Autodesk Inventor part; units mm, degrees
(part 2 of 2)
sketch "Эскиз17" plane through (97.4, -95.275, 2.1) normal (1, 0, 0) x (0, 0, -1)
  line L0 (-33.4467, 33.4271) -> (-33.4467, 22.4297) construction
  line L1 (-33.4467, 22.4297) -> (-36.1893, 22.4297) construction
  line L2 (-36.1893, 22.4297) -> (-36.1893, 33.4271) construction
  line L3 (-36.1893, 33.4271) -> (-33.4467, 33.4271) construction
  line L4 (-30.2454, 64.7817) -> (-30.2454, 44.3238) construction
  line L5 (-30.2454, 44.3238) -> (-33.7846, 44.3238) construction
  line L6 (-33.7846, 44.3238) -> (-33.7846, 64.7817) construction
  line L7 (-33.7846, 64.7817) -> (-30.2454, 64.7817) construction
  spline S0 degree 2 poles (-31.5525, 64.6293) (-31.1714, 64.6293) (-30.9123, 64.515) knots 0 0 0 1 1 1
  spline S1 degree 2 poles (-30.9123, 64.515) (-30.7218, 64.4292) (-30.4169, 64.1339) (-30.3445, 63.9586) knots 0 0 0 1 2 2 2
  spline S2 degree 2 poles (-30.3445, 63.9586) (-30.2454, 63.7261) (-30.2454, 63.4193) knots 0 0 0 1 1 1
  spline S3 degree 2 poles (-30.2454, 63.4193) (-30.2454, 62.8667) (-30.9314, 62.2036) (-31.5411, 62.2036) knots 0 0 0 1 2 2 2
  spline S4 degree 2 poles (-31.5411, 62.2036) (-32.1452, 62.2036) (-32.8292, 62.8629) (-32.8292, 63.4136) knots 0 0 0 1 2 2 2
  spline S5 degree 2 poles (-32.8292, 63.4136) (-32.8292, 63.97) (-32.149, 64.6293) (-31.5525, 64.6293) knots 0 0 0 1 2 2 2
  spline S6 degree 2 poles (-31.5354, 64.1091) (-31.9603, 64.1091) (-32.3986, 63.7166) (-32.3986, 63.4136) knots 0 0 0 1 2 2 2
  spline S7 degree 2 poles (-32.3986, 63.4136) (-32.3986, 63.1106) (-31.9641, 62.7238) (-31.5297, 62.7238) knots 0 0 0 1 2 2 2
  spline S8 degree 2 poles (-31.5297, 62.7238) (-31.099, 62.7238) (-30.676, 63.1011) (-30.676, 63.4136) knots 0 0 0 1 2 2 2
  spline S9 degree 2 poles (-30.676, 63.4136) (-30.676, 63.7261) (-31.1048, 64.1091) (-31.5354, 64.1091) knots 0 0 0 1 2 2 2
  line L8 (-30.9752, 61.8282) -> (-30.9752, 61.3804)
  line L9 (-30.9752, 61.3804) -> (-31.242, 61.3804)
  spline S10 degree 2 poles (-31.242, 61.3804) (-31.1048, 61.2928) (-30.9352, 60.9974) (-30.9352, 60.8164) knots 0 0 0 1 2 2 2
  spline S11 degree 2 poles (-30.9352, 60.8164) (-30.9352, 60.5001) (-31.4287, 60.0599) (-31.8708, 60.0599) knots 0 0 0 1 2 2 2
  spline S12 degree 2 poles (-31.8708, 60.0599) (-32.3243, 60.0599) (-32.8273, 60.5039) (-32.8273, 60.8183) knots 0 0 0 1 2 2 2
  spline S13 degree 2 poles (-32.8273, 60.8183) (-32.8273, 60.9688) (-32.7073, 61.2127) (-32.5625, 61.348) knots 0 0 0 1 2 2 2
  line L10 (-32.5625, 61.348) -> (-33.4771, 61.348)
  line L11 (-33.4771, 61.348) -> (-33.4771, 61.8282)
  line L12 (-33.4771, 61.8282) -> (-30.9752, 61.8282)
  spline S14 degree 2 poles (-31.8498, 61.3557) (-32.1547, 61.3557) (-32.4462, 61.1118) (-32.4462, 60.9384) knots 0 0 0 1 2 2 2
  spline S15 degree 2 poles (-32.4462, 60.9384) (-32.4462, 60.7707) (-32.1795, 60.5477) (-31.8746, 60.5477) knots 0 0 0 1 2 2 2
  spline S16 degree 2 poles (-31.8746, 60.5477) (-31.5907, 60.5477) (-31.3144, 60.7764) (-31.3144, 60.946) knots 0 0 0 1 2 2 2
  spline S17 degree 2 poles (-31.3144, 60.946) (-31.3144, 61.1232) (-31.5849, 61.3557) (-31.8498, 61.3557) knots 0 0 0 1 2 2 2
  line L13 (-32.7873, 59.6788) -> (-30.9752, 59.6788)
  line L14 (-30.9752, 59.6788) -> (-30.9752, 59.1986)
  line L15 (-30.9752, 59.1986) -> (-32.7873, 59.1986)
  line L16 (-32.7873, 59.1986) -> (-32.7873, 59.6788)
  line L17 (-30.7313, 59.6788) -> (-30.2873, 59.6788)
  line L18 (-30.2873, 59.6788) -> (-30.2873, 59.1986)
  line L19 (-30.2873, 59.1986) -> (-30.7313, 59.1986)
  line L20 (-30.7313, 59.1986) -> (-30.7313, 59.6788)
  line L21 (-31.5106, 57.1331) -> (-31.5964, 57.6057)
  spline S18 degree 2 poles (-31.5964, 57.6057) (-31.4554, 57.6285) (-31.3125, 57.7981) (-31.3125, 57.9334) knots 0 0 0 1 2 2 2
  spline S19 degree 2 poles (-31.3125, 57.9334) (-31.3125, 58.1106) (-31.5602, 58.324) (-31.8498, 58.324) knots 0 0 0 1 2 2 2
  spline S20 degree 2 poles (-31.8498, 58.324) (-32.1718, 58.324) (-32.4367, 58.1068) (-32.4367, 57.9258) knots 0 0 0 1 2 2 2
  spline S21 degree 2 poles (-32.4367, 57.9258) (-32.4367, 57.7886) (-32.2804, 57.6152) (-32.0918, 57.579) knots 0 0 0 1 2 2 2
  line L22 (-32.0918, 57.579) -> (-32.1718, 57.1083)
  spline S22 degree 2 poles (-32.1718, 57.1083) (-32.4958, 57.1807) (-32.8273, 57.598) (-32.8273, 57.9467) knots 0 0 0 1 2 2 2
  spline S23 degree 2 poles (-32.8273, 57.9467) (-32.8273, 58.3431) (-32.3262, 58.8156) (-31.8822, 58.8156) knots 0 0 0 1 2 2 2
  spline S24 degree 2 poles (-31.8822, 58.8156) (-31.4344, 58.8156) (-30.9352, 58.3431) (-30.9352, 57.9391) knots 0 0 0 1 2 2 2
  spline S25 degree 2 poles (-30.9352, 57.9391) (-30.9352, 57.6076) (-31.2191, 57.2188) (-31.5106, 57.1331) knots 0 0 0 1 2 2 2
  line L23 (-31.5278, 56.4109) -> (-31.4496, 56.8454)
  spline S26 degree 2 poles (-31.4496, 56.8454) (-31.1867, 56.7711) (-30.9352, 56.4128) (-30.9352, 56.0603) knots 0 0 0 1 2 2 2
  spline S27 degree 2 poles (-30.9352, 56.0603) (-30.9352, 55.7383) (-31.0876, 55.4239) (-31.3201, 55.2962) (-31.6326, 55.2962) knots 0 0 0 1 2 3 3 3
  line L24 (-31.6326, 55.2962) -> (-32.1928, 55.3038)
  spline S28 degree 2 poles (-32.1928, 55.3038) (-32.431, 55.3038) (-32.6577, 55.2581) (-32.7873, 55.1952) knots 0 0 0 1 2 2 2
  line L25 (-32.7873, 55.1952) -> (-32.7873, 55.6697)
  spline S29 degree 2 poles (-32.7873, 55.6697) (-32.7397, 55.6887) (-32.6463, 55.7154) knots 0 0 0 1 1 1
  spline S30 degree 2 poles (-32.6463, 55.7154) (-32.6025, 55.7268) (-32.5891, 55.7326) knots 0 0 0 1 1 1
  spline S31 degree 2 poles (-32.5891, 55.7326) (-32.7073, 55.8545) (-32.8273, 56.1346) (-32.8273, 56.2928) knots 0 0 0 1 2 2 2
  spline S32 degree 2 poles (-32.8273, 56.2928) (-32.8273, 56.5729) (-32.5243, 56.8949) (-32.2919, 56.8949) knots 0 0 0 1 2 2 2
  spline S33 degree 2 poles (-32.2919, 56.8949) (-32.1375, 56.8949) (-31.8974, 56.7482) (-31.7698, 56.4833) (-31.7221, 56.2337) knots 0 0 0 1 2 3 3 3
  spline S34 degree 2 poles (-31.7221, 56.2337) (-31.6593, 55.8983) (-31.604, 55.7688) knots 0 0 0 1 1 1
  line L26 (-31.604, 55.7688) -> (-31.5564, 55.7688)
  spline S35 degree 2 poles (-31.5564, 55.7688) (-31.4192, 55.7688) (-31.301, 55.906) (-31.301, 56.0946) knots 0 0 0 1 2 2 2
  spline S36 degree 2 poles (-31.301, 56.0946) (-31.301, 56.2223) (-31.402, 56.3671) (-31.5278, 56.4109) knots 0 0 0 1 2 2 2
  spline S37 degree 2 poles (-31.9165, 55.7688) (-31.947, 55.8602) (-32.0327, 56.2604) (-32.0727, 56.3214) knots 0 0 0 1 2 2 2
  spline S38 degree 2 poles (-32.0727, 56.3214) (-32.1394, 56.4147) (-32.2423, 56.4147) knots 0 0 0 1 1 1
  spline S39 degree 2 poles (-32.2423, 56.4147) (-32.3433, 56.4147) (-32.49, 56.2642) (-32.49, 56.148) knots 0 0 0 1 2 2 2
  spline S40 degree 2 poles (-32.49, 56.148) (-32.49, 56.0184) (-32.4043, 55.9022) knots 0 0 0 1 1 1
  spline S41 degree 2 poles (-32.4043, 55.9022) (-32.3395, 55.8145) (-32.2461, 55.7878) knots 0 0 0 1 1 1
  spline S42 degree 2 poles (-32.2461, 55.7878) (-32.1852, 55.7688) (-32.0118, 55.7688) knots 0 0 0 1 1 1
  line L27 (-32.0118, 55.7688) -> (-31.9165, 55.7688)
  line L28 (-32.7873, 54.8256) -> (-30.2873, 54.8256)
  line L29 (-30.2873, 54.8256) -> (-30.2873, 54.3454)
  line L30 (-30.2873, 54.3454) -> (-32.7873, 54.3454)
  line L31 (-32.7873, 54.3454) -> (-32.7873, 54.8256)
  line L32 (-32.7873, 52.8858) -> (-30.9752, 52.8858)
  line L33 (-30.9752, 52.8858) -> (-30.9752, 52.4056)
  line L34 (-30.9752, 52.4056) -> (-32.7873, 52.4056)
  line L35 (-32.7873, 52.4056) -> (-32.7873, 52.8858)
  line L36 (-30.7313, 52.8858) -> (-30.2873, 52.8858)
  line L37 (-30.2873, 52.8858) -> (-30.2873, 52.4056)
  line L38 (-30.2873, 52.4056) -> (-30.7313, 52.4056)
  line L39 (-30.7313, 52.4056) -> (-30.7313, 52.8858)
  line L40 (-32.7873, 50.2695) -> (-32.7873, 50.7497)
  line L41 (-32.7873, 50.7497) -> (-31.8631, 50.7497)
  spline S43 degree 2 poles (-31.8631, 50.7497) (-31.5697, 50.7497) (-31.3963, 50.8107) (-31.301, 50.9498) (-31.301, 51.047) knots 0 0 0 1 2 3 3 3
  spline S44 degree 2 poles (-31.301, 51.047) (-31.301, 51.1708) (-31.4382, 51.369) (-31.6631, 51.4414) (-31.966, 51.4414) knots 0 0 0 1 2 3 3 3
  line L42 (-31.966, 51.4414) -> (-32.7873, 51.4414)
  line L43 (-32.7873, 51.4414) -> (-32.7873, 51.9216)
  line L44 (-32.7873, 51.9216) -> (-30.9752, 51.9216)
  line L45 (-30.9752, 51.9216) -> (-30.9752, 51.4757)
  line L46 (-30.9752, 51.4757) -> (-31.242, 51.4757)
  spline S45 degree 2 poles (-31.242, 51.4757) (-30.9352, 51.2394) (-30.9352, 50.8793) knots 0 0 0 1 1 1
  spline S46 degree 2 poles (-30.9352, 50.8793) (-30.9352, 50.7192) (-31.0495, 50.4563) (-31.2267, 50.3229) (-31.4516, 50.2695) (-31.6612, 50.2695) knots 0 0 0 1 2 3 4 4 4
  line L47 (-31.6612, 50.2695) -> (-32.7873, 50.2695)
  line L48 (-30.9752, 49.797) -> (-30.9752, 49.3492)
  line L49 (-30.9752, 49.3492) -> (-31.242, 49.3492)
  spline S47 degree 2 poles (-31.242, 49.3492) (-31.1048, 49.2615) (-30.9352, 48.9662) (-30.9352, 48.7852) knots 0 0 0 1 2 2 2
  spline S48 degree 2 poles (-30.9352, 48.7852) (-30.9352, 48.4688) (-31.4287, 48.0287) (-31.8708, 48.0287) knots 0 0 0 1 2 2 2
  spline S49 degree 2 poles (-31.8708, 48.0287) (-32.3243, 48.0287) (-32.8273, 48.4727) (-32.8273, 48.7871) knots 0 0 0 1 2 2 2
  spline S50 degree 2 poles (-32.8273, 48.7871) (-32.8273, 48.9376) (-32.7073, 49.1815) (-32.5625, 49.3168) knots 0 0 0 1 2 2 2
  line L50 (-32.5625, 49.3168) -> (-33.4771, 49.3168)
  line L51 (-33.4771, 49.3168) -> (-33.4771, 49.797)
  line L52 (-33.4771, 49.797) -> (-30.9752, 49.797)
  spline S51 degree 2 poles (-31.8498, 49.3244) (-32.1547, 49.3244) (-32.4462, 49.0805) (-32.4462, 48.9071) knots 0 0 0 1 2 2 2
  spline S52 degree 2 poles (-32.4462, 48.9071) (-32.4462, 48.7394) (-32.1795, 48.5165) (-31.8746, 48.5165) knots 0 0 0 1 2 2 2
  spline S53 degree 2 poles (-31.8746, 48.5165) (-31.5907, 48.5165) (-31.3144, 48.7451) (-31.3144, 48.9147) knots 0 0 0 1 2 2 2
  spline S54 degree 2 poles (-31.3144, 48.9147) (-31.3144, 49.0919) (-31.5849, 49.3244) (-31.8498, 49.3244) knots 0 0 0 1 2 2 2
  line L53 (-32.7873, 46.4566) -> (-32.5167, 46.4566)
  spline S55 degree 2 poles (-32.5167, 46.4566) (-32.6615, 46.5557) (-32.8273, 46.8778) (-32.8273, 47.0569) knots 0 0 0 1 2 2 2
  spline S56 degree 2 poles (-32.8273, 47.0569) (-32.8273, 47.2398) (-32.6673, 47.5294) (-32.3776, 47.659) (-32.1204, 47.659) knots 0 0 0 1 2 3 3 3
  line L54 (-32.1204, 47.659) -> (-30.9752, 47.659)
  line L55 (-30.9752, 47.659) -> (-30.9752, 47.1788)
  line L56 (-30.9752, 47.1788) -> (-31.8079, 47.1788)
  spline S57 degree 2 poles (-31.8079, 47.1788) (-32.189, 47.1788) (-32.3605, 47.1255) (-32.4615, 46.9864) (-32.4615, 46.8797) knots 0 0 0 1 2 3 3 3
  spline S58 degree 2 poles (-32.4615, 46.8797) (-32.4615, 46.7558) (-32.3262, 46.5634) (-32.128, 46.4909) (-31.7393, 46.4909) knots 0 0 0 1 2 3 3 3
  line L57 (-31.7393, 46.4909) -> (-30.9752, 46.4909)
  line L58 (-30.9752, 46.4909) -> (-30.9752, 46.0108)
  line L59 (-30.9752, 46.0108) -> (-32.7873, 46.0108)
  line L60 (-32.7873, 46.0108) -> (-32.7873, 46.4566)
  line L61 (-30.9752, 44.6845) -> (-31.3563, 44.6845)
  line L62 (-31.3563, 44.6845) -> (-31.3563, 45.0123)
  line L63 (-31.3563, 45.0123) -> (-32.0861, 45.0123)
  spline S59 degree 2 poles (-32.0861, 45.0123) (-32.3071, 45.0123) (-32.3814, 44.9932) (-32.4291, 44.9265) (-32.4291, 44.8789) knots 0 0 0 1 2 3 3 3
  spline S60 degree 2 poles (-32.4291, 44.8789) (-32.4291, 44.8122) (-32.3833, 44.6845) knots 0 0 0 1 1 1
  line L64 (-32.3833, 44.6845) -> (-32.7549, 44.6445)
  spline S61 degree 2 poles (-32.7549, 44.6445) (-32.8273, 44.8122) (-32.8273, 45.0237) knots 0 0 0 1 1 1
  spline S62 degree 2 poles (-32.8273, 45.0237) (-32.8273, 45.1533) (-32.7397, 45.361) (-32.6025, 45.4582) (-32.4843, 45.4772) knots 0 0 0 1 2 3 3 3
  spline S63 degree 2 poles (-32.4843, 45.4772) (-32.4005, 45.4925) (-32.1471, 45.4925) knots 0 0 0 1 1 1
  line L65 (-32.1471, 45.4925) -> (-31.3563, 45.4925)
  line L66 (-31.3563, 45.4925) -> (-31.3563, 45.7116)
  line L67 (-31.3563, 45.7116) -> (-30.9752, 45.7116)
  line L68 (-30.9752, 45.7116) -> (-30.9752, 45.4925)
  line L69 (-30.9752, 45.4925) -> (-30.615, 45.4925)
  line L70 (-30.615, 45.4925) -> (-30.333, 45.0123)
  line L71 (-30.333, 45.0123) -> (-30.9752, 45.0123)
  line L72 (-30.9752, 45.0123) -> (-30.9752, 44.6845)
  line L73 (-35.1731, 33.3014) -> (-35.1255, 32.8097)
  spline S64 degree 2 poles (-35.1255, 32.8097) (-35.3732, 32.7659) (-35.6057, 32.4934) (-35.6057, 32.2648) knots 0 0 0 1 2 2 2
  spline S65 degree 2 poles (-35.6057, 32.2648) (-35.6057, 32.0209) (-35.3999, 31.7732) (-35.2608, 31.7732) knots 0 0 0 1 2 2 2
  spline S66 degree 2 poles (-35.2608, 31.7732) (-35.1712, 31.7732) (-35.0474, 31.878) (-35.0016, 32.0075) knots 0 0 0 1 2 2 2
  spline S67 degree 2 poles (-35.0016, 32.0075) (-34.9711, 32.0952) (-34.893, 32.4115) knots 0 0 0 1 1 1
  spline S68 degree 2 poles (-34.893, 32.4115) (-34.792, 32.8174) (-34.6453, 32.9812) knots 0 0 0 1 1 1
  spline S69 degree 2 poles (-34.6453, 32.9812) (-34.4395, 33.2118) (-34.1442, 33.2118) knots 0 0 0 1 1 1
  spline S70 degree 2 poles (-34.1442, 33.2118) (-33.9517, 33.2118) (-33.6201, 32.9946) (-33.4467, 32.5868) (-33.4467, 32.2991) knots 0 0 0 1 2 3 3 3
  spline S71 degree 2 poles (-33.4467, 32.2991) (-33.4467, 31.8284) (-33.8583, 31.352) (-34.2032, 31.3406) knots 0 0 0 1 2 2 2
  line L74 (-34.2032, 31.3406) -> (-34.2261, 31.8456)
  spline S72 degree 2 poles (-34.2261, 31.8456) (-34.0336, 31.878) (-33.864, 32.0914) (-33.864, 32.3048) knots 0 0 0 1 2 2 2
  spline S73 degree 2 poles (-33.864, 32.3048) (-33.864, 32.5258) (-33.9536, 32.6497) knots 0 0 0 1 1 1
  spline S74 degree 2 poles (-33.9536, 32.6497) (-34.0127, 32.7297) (-34.1099, 32.7297) knots 0 0 0 1 1 1
  spline S75 degree 2 poles (-34.1099, 32.7297) (-34.1975, 32.7297) (-34.2623, 32.6554) knots 0 0 0 1 1 1
  spline S76 degree 2 poles (-34.2623, 32.6554) (-34.3423, 32.5582) (-34.5157, 31.8208) (-34.7006, 31.4683) (-35.0226, 31.2682) (-35.2608, 31.2682) knots 0 0 0 1 2 3 4 4 4
  spline S77 degree 2 poles (-35.2608, 31.2682) (-35.4742, 31.2682) (-35.8496, 31.5064) (-36.0325, 31.9427) (-36.0325, 32.2686) knots 0 0 0 1 2 3 3 3
  spline S78 degree 2 poles (-36.0325, 32.2686) (-36.0325, 32.7431) (-35.5942, 33.2518) (-35.1731, 33.3014) knots 0 0 0 1 2 2 2
  line L75 (-34.1765, 30.0163) -> (-34.5576, 30.0163)
  line L76 (-34.5576, 30.0163) -> (-34.5576, 30.344)
  line L77 (-34.5576, 30.344) -> (-35.2874, 30.344)
  spline S79 degree 2 poles (-35.2874, 30.344) (-35.5085, 30.344) (-35.5828, 30.325) (-35.6304, 30.2583) (-35.6304, 30.2107) knots 0 0 0 1 2 3 3 3
  spline S80 degree 2 poles (-35.6304, 30.2107) (-35.6304, 30.144) (-35.5847, 30.0163) knots 0 0 0 1 1 1
  line L78 (-35.5847, 30.0163) -> (-35.9563, 29.9763)
  spline S81 degree 2 poles (-35.9563, 29.9763) (-36.0287, 30.144) (-36.0287, 30.3555) knots 0 0 0 1 1 1
  spline S82 degree 2 poles (-36.0287, 30.3555) (-36.0287, 30.485) (-35.941, 30.6927) (-35.8038, 30.7899) (-35.6857, 30.809) knots 0 0 0 1 2 3 3 3
  spline S83 degree 2 poles (-35.6857, 30.809) (-35.6019, 30.8242) (-35.3484, 30.8242) knots 0 0 0 1 1 1
  line L79 (-35.3484, 30.8242) -> (-34.5576, 30.8242)
  line L80 (-34.5576, 30.8242) -> (-34.5576, 31.0434)
  line L81 (-34.5576, 31.0434) -> (-34.1765, 31.0434)
  line L82 (-34.1765, 31.0434) -> (-34.1765, 30.8242)
  line L83 (-34.1765, 30.8242) -> (-33.8164, 30.8242)
  line L84 (-33.8164, 30.8242) -> (-33.5344, 30.344)
  line L85 (-33.5344, 30.344) -> (-34.1765, 30.344)
  line L86 (-34.1765, 30.344) -> (-34.1765, 30.0163)
  line L87 (-34.7291, 29.3265) -> (-34.651, 29.761)
  spline S84 degree 2 poles (-34.651, 29.761) (-34.3881, 29.6866) (-34.1365, 29.3284) (-34.1365, 28.9759) knots 0 0 0 1 2 2 2
  spline S85 degree 2 poles (-34.1365, 28.9759) (-34.1365, 28.6539) (-34.289, 28.3395) (-34.5214, 28.2118) (-34.8339, 28.2118) knots 0 0 0 1 2 3 3 3
  line L88 (-34.8339, 28.2118) -> (-35.3942, 28.2194)
  spline S86 degree 2 poles (-35.3942, 28.2194) (-35.6323, 28.2194) (-35.8591, 28.1737) (-35.9887, 28.1108) knots 0 0 0 1 2 2 2
  line L89 (-35.9887, 28.1108) -> (-35.9887, 28.5853)
  spline S87 degree 2 poles (-35.9887, 28.5853) (-35.941, 28.6043) (-35.8477, 28.631) knots 0 0 0 1 1 1
  spline S88 degree 2 poles (-35.8477, 28.631) (-35.8038, 28.6424) (-35.7905, 28.6482) knots 0 0 0 1 1 1
  spline S89 degree 2 poles (-35.7905, 28.6482) (-35.9086, 28.7701) (-36.0287, 29.0502) (-36.0287, 29.2084) knots 0 0 0 1 2 2 2
  spline S90 degree 2 poles (-36.0287, 29.2084) (-36.0287, 29.4885) (-35.7257, 29.8105) (-35.4932, 29.8105) knots 0 0 0 1 2 2 2
  spline S91 degree 2 poles (-35.4932, 29.8105) (-35.3389, 29.8105) (-35.0988, 29.6638) (-34.9711, 29.3989) (-34.9235, 29.1493) knots 0 0 0 1 2 3 3 3
  spline S92 degree 2 poles (-34.9235, 29.1493) (-34.8606, 28.8139) (-34.8054, 28.6844) knots 0 0 0 1 1 1
  line L90 (-34.8054, 28.6844) -> (-34.7577, 28.6844)
  spline S93 degree 2 poles (-34.7577, 28.6844) (-34.6205, 28.6844) (-34.5024, 28.8216) (-34.5024, 29.0102) knots 0 0 0 1 2 2 2
  spline S94 degree 2 poles (-34.5024, 29.0102) (-34.5024, 29.1379) (-34.6034, 29.2827) (-34.7291, 29.3265) knots 0 0 0 1 2 2 2
  spline S95 degree 2 poles (-35.1179, 28.6844) (-35.1483, 28.7758) (-35.2341, 29.176) (-35.2741, 29.237) knots 0 0 0 1 2 2 2
  spline S96 degree 2 poles (-35.2741, 29.237) (-35.3408, 29.3303) (-35.4437, 29.3303) knots 0 0 0 1 1 1
  spline S97 degree 2 poles (-35.4437, 29.3303) (-35.5447, 29.3303) (-35.6914, 29.1798) (-35.6914, 29.0636) knots 0 0 0 1 2 2 2
  spline S98 degree 2 poles (-35.6914, 29.0636) (-35.6914, 28.934) (-35.6057, 28.8177) knots 0 0 0 1 1 1
  spline S99 degree 2 poles (-35.6057, 28.8177) (-35.5409, 28.7301) (-35.4475, 28.7034) knots 0 0 0 1 1 1
  spline S100 degree 2 poles (-35.4475, 28.7034) (-35.3865, 28.6844) (-35.2131, 28.6844) knots 0 0 0 1 1 1
  line L91 (-35.2131, 28.6844) -> (-35.1179, 28.6844)
  line L92 (-34.1765, 26.9123) -> (-34.5576, 26.9123)
  line L93 (-34.5576, 26.9123) -> (-34.5576, 27.24)
  line L94 (-34.5576, 27.24) -> (-35.2874, 27.24)
  spline S101 degree 2 poles (-35.2874, 27.24) (-35.5085, 27.24) (-35.5828, 27.2209) (-35.6304, 27.1543) (-35.6304, 27.1066) knots 0 0 0 1 2 3 3 3
  spline S102 degree 2 poles (-35.6304, 27.1066) (-35.6304, 27.0399) (-35.5847, 26.9123) knots 0 0 0 1 1 1
  line L95 (-35.5847, 26.9123) -> (-35.9563, 26.8722)
  spline S103 degree 2 poles (-35.9563, 26.8722) (-36.0287, 27.0399) (-36.0287, 27.2514) knots 0 0 0 1 1 1
  spline S104 degree 2 poles (-36.0287, 27.2514) (-36.0287, 27.381) (-35.941, 27.5887) (-35.8038, 27.6859) (-35.6857, 27.7049) knots 0 0 0 1 2 3 3 3
  spline S105 degree 2 poles (-35.6857, 27.7049) (-35.6019, 27.7202) (-35.3484, 27.7202) knots 0 0 0 1 1 1
  line L96 (-35.3484, 27.7202) -> (-34.5576, 27.7202)
  line L97 (-34.5576, 27.7202) -> (-34.5576, 27.9393)
  line L98 (-34.5576, 27.9393) -> (-34.1765, 27.9393)
  line L99 (-34.1765, 27.9393) -> (-34.1765, 27.7202)
  line L100 (-34.1765, 27.7202) -> (-33.8164, 27.7202)
  line L101 (-33.8164, 27.7202) -> (-33.5344, 27.24)
  line L102 (-33.5344, 27.24) -> (-34.1765, 27.24)
  line L103 (-34.1765, 27.24) -> (-34.1765, 26.9123)
  line L104 (-35.9887, 25.3879) -> (-35.7181, 25.3879)
  spline S106 degree 2 poles (-35.7181, 25.3879) (-35.8629, 25.487) (-36.0287, 25.809) (-36.0287, 25.9881) knots 0 0 0 1 2 2 2
  spline S107 degree 2 poles (-36.0287, 25.9881) (-36.0287, 26.171) (-35.8686, 26.4607) (-35.579, 26.5902) (-35.3217, 26.5902) knots 0 0 0 1 2 3 3 3
  line L105 (-35.3217, 26.5902) -> (-34.1765, 26.5902)
  line L106 (-34.1765, 26.5902) -> (-34.1765, 26.11)
  line L107 (-34.1765, 26.11) -> (-35.0092, 26.11)
  spline S108 degree 2 poles (-35.0092, 26.11) (-35.3903, 26.11) (-35.5618, 26.0567) (-35.6628, 25.9176) (-35.6628, 25.8109) knots 0 0 0 1 2 3 3 3
  spline S109 degree 2 poles (-35.6628, 25.8109) (-35.6628, 25.687) (-35.5275, 25.4946) (-35.3294, 25.4222) (-34.9406, 25.4222) knots 0 0 0 1 2 3 3 3
  line L108 (-34.9406, 25.4222) -> (-34.1765, 25.4222)
  line L109 (-34.1765, 25.4222) -> (-34.1765, 24.942)
  line L110 (-34.1765, 24.942) -> (-35.9887, 24.942)
  line L111 (-35.9887, 24.942) -> (-35.9887, 25.3879)
  line L112 (-35.4704, 24.6142) -> (-35.398, 24.1341)
  spline S110 degree 2 poles (-35.398, 24.1341) (-35.5371, 24.1036) (-35.6819, 23.9149) (-35.6819, 23.7472) knots 0 0 0 1 2 2 2
  spline S111 degree 2 poles (-35.6819, 23.7472) (-35.6819, 23.5605) (-35.6133, 23.4671) knots 0 0 0 1 1 1
  spline S112 degree 2 poles (-35.6133, 23.4671) (-35.5656, 23.4043) (-35.4856, 23.4043) knots 0 0 0 1 1 1
  spline S113 degree 2 poles (-35.4856, 23.4043) (-35.4323, 23.4043) (-35.3961, 23.4386) knots 0 0 0 1 1 1
  spline S114 degree 2 poles (-35.3961, 23.4386) (-35.3618, 23.4748) (-35.3332, 23.5986) knots 0 0 0 1 1 1
  spline S115 degree 2 poles (-35.3332, 23.5986) (-35.2055, 24.1779) (-35.0988, 24.3322) knots 0 0 0 1 1 1
  spline S116 degree 2 poles (-35.0988, 24.3322) (-34.9521, 24.5475) (-34.6929, 24.5475) knots 0 0 0 1 1 1
  spline S117 degree 2 poles (-34.6929, 24.5475) (-34.4567, 24.5475) (-34.1365, 24.176) (-34.1365, 23.7854) knots 0 0 0 1 2 2 2
  spline S118 degree 2 poles (-34.1365, 23.7854) (-34.1365, 23.4138) (-34.3785, 23.0536) (-34.6167, 22.985) knots 0 0 0 1 2 2 2
  line L113 (-34.6167, 22.985) -> (-34.7006, 23.4366)
  spline S119 degree 2 poles (-34.7006, 23.4366) (-34.5939, 23.4652) (-34.4814, 23.6272) (-34.4814, 23.7777) knots 0 0 0 1 2 2 2
  spline S120 degree 2 poles (-34.4814, 23.7777) (-34.4814, 23.9664) (-34.5348, 24.0464) knots 0 0 0 1 1 1
  spline S121 degree 2 poles (-34.5348, 24.0464) (-34.571, 24.1017) (-34.632, 24.1017) knots 0 0 0 1 1 1
  spline S122 degree 2 poles (-34.632, 24.1017) (-34.6815, 24.1017) (-34.7177, 24.054) knots 0 0 0 1 1 1
  spline S123 degree 2 poles (-34.7177, 24.054) (-34.7653, 23.9892) (-34.9387, 23.2251) (-35.0664, 23.0746) knots 0 0 0 1 2 2 2
  spline S124 degree 2 poles (-35.0664, 23.0746) (-35.1941, 22.9241) (-35.4227, 22.9241) knots 0 0 0 1 1 1
  spline S125 degree 2 poles (-35.4227, 22.9241) (-35.6705, 22.9241) (-36.0287, 23.3395) (-36.0287, 23.7472) knots 0 0 0 1 2 2 2
  spline S126 degree 2 poles (-36.0287, 23.7472) (-36.0287, 24.1169) (-35.7276, 24.5475) (-35.4704, 24.6142) knots 0 0 0 1 2 2 2
  point P0 (2.1, 95.275)
  constraints: 4 other
emboss "Рельеф1" sketch "Эскиз17" operation cut depth 0.6 direction (-1, 0, 0)
sketch "Эскиз4" plane through (0, 0, 53.6) normal (0, 0, 1) x (1, 0, 0)
  circle A0 centre (1.5, -93.775) radius 2.3 projected
  circle A1 centre (1.5, -6.375) radius 2.3 projected
  circle A2 centre (88.9, -6.375) radius 2.3 projected
  circle A3 centre (88.9, -93.775) radius 2.3 projected
  circle A4 centre (1.5, -93.775) radius 6
  circle A5 centre (1.5, -6.375) radius 6
  circle A6 centre (88.9, -93.775) radius 6
  circle A7 centre (88.9, -6.375) radius 6
  circle A8 centre (88.9, -6.375) radius 4.6
  circle A9 centre (88.9, -93.775) radius 4.6
  circle A10 centre (1.5, -93.775) radius 4.6
  circle A11 centre (1.5, -6.375) radius 4.6
  point P0 (0, 0)
  dimension "d12" = 12
  dimension "d13" = 12
  dimension "d14" = 12
  dimension "d15" = 12
  dimension "d16" = 1.4
  dimension "d17" = 1.4
  dimension "d18" = 1.4
  dimension "d19" = 1.4
  constraints: 8 centre point, 4 coincident
  measures "d12" diameter of A4
  measures "d13" diameter of A5
  measures "d14" diameter of A6
  measures "d15" diameter of A7
  measures "d16" radial gap between concentric circles of A7 A8
  measures "d17" radial gap between concentric circles of A6 A9
  measures "d18" radial gap between concentric circles of A4 A10
  measures "d19" radial gap between concentric circles of A5 A11
extrude "Выдавливание15" cut sketch "Эскиз4" against normal blind 1 contours A4 | A5 | A6 | A7
sketch "Эскиз18" plane through (0, 0, 53.6) normal (0, 0, 1) x (1, 0, 0)
  circle A0 centre (1.5, -93.775) radius 4.6 projected
  circle A1 centre (1.5, -93.775) radius 6 projected
  circle A2 centre (88.9, -93.775) radius 4.6 projected
  circle A3 centre (88.9, -93.775) radius 6 projected
  circle A4 centre (88.9, -6.375) radius 4.6 projected
  circle A5 centre (88.9, -6.375) radius 6 projected
  circle A6 centre (1.5, -6.375) radius 4.6 projected
  circle A7 centre (1.5, -6.375) radius 6 projected
  circle A8 centre (1.5, -93.775) radius 6.1
  circle A9 centre (1.5, -93.775) radius 4.5
  circle A10 centre (1.5, -6.375) radius 6.1
  circle A11 centre (1.5, -6.375) radius 4.5
  circle A12 centre (88.9, -6.375) radius 4.5
  circle A13 centre (88.9, -6.375) radius 6.1
  circle A14 centre (88.9, -93.775) radius 6.1
  circle A15 centre (88.9, -93.775) radius 4.5
  point P0 (0, 0)
  dimension "d242" = 0.1
  dimension "d243" = 0.1
  dimension "d244" = 0.1
  dimension "d245" = 0.1
  dimension "d246" = 0.1
  dimension "d247" = 0.1
  dimension "d248" = 0.1
  dimension "d249" = 0.1
  constraints: 8 centre point
  measures "d242" radial gap between concentric circles of A1 A8
  measures "d243" radial gap between concentric circles of A0 A9
  measures "d244" radial gap between concentric circles of A7 A10
  measures "d245" radial gap between concentric circles of A6 A11
  measures "d246" radial gap between concentric circles of A4 A12
  measures "d247" radial gap between concentric circles of A5 A13
  measures "d248" radial gap between concentric circles of A3 A14
  measures "d249" radial gap between concentric circles of A2 A15
extrude "Выдавливание16" cut sketch "Эскиз18" against normal up to surface (1 mm away) contours A0 | A1 | A2 | A3 | A4 | A5 | A6 | A7 | A8 | A10 | A13 | A14
sketch "Эскиз19" plane through (0, 0, 53.6) normal (0, 0, 1) x (1, 0, 0)
  circle A0 centre (88.9, -93.775) radius 4
  circle A1 centre (88.9, -6.375) radius 3.5 projected
  circle A2 centre (88.9, -6.375) radius 4
  circle A3 centre (1.5, -6.375) radius 4
  circle A4 centre (1.5, -93.775) radius 4
  point P0 (0, 0)
  dimension "d252" = 8
  dimension "d253" = 8
  dimension "d254" = 8
  dimension "d255" = 8
  constraints: 4 centre point, 4 coincident
  measures "d252" diameter of A0
  measures "d253" diameter of A2
  measures "d254" diameter of A3
  measures "d255" diameter of A4
extrude "Выдавливание17" cut sketch "Эскиз19" against normal up to surface (39 mm away) contours A0 | A1 | A2 | A3 | A4
